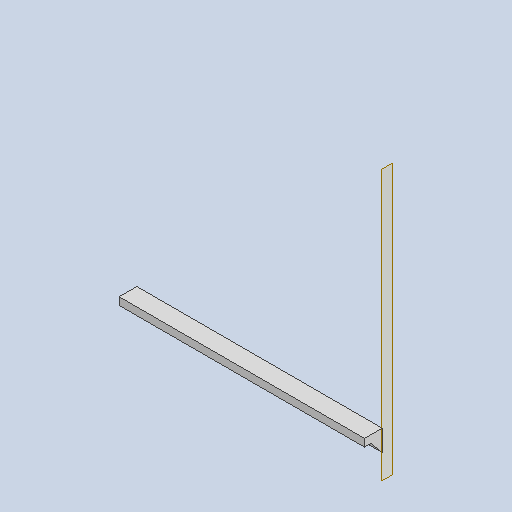
# Autodesk Inventor part: PlasticBody
Saved by Autodesk Inventor 2023 (Build 270158000, 158)
## iProperties
Created: 2024-03-04
Part Number: PlasticBody
Material: Generic
Document SubType Name: Modeling
Designer: pavel
Density: 1 g/cm^3
Appearance: Default
Author: pavel
Autodesk Inventor part; units mm, degrees
ref_plane "YZ Plane" through (0, 0, 0) normal (1, 0, 0) x (0, 1, 0)
ref_plane "XZ Plane" through (0, 0, 0) normal (0, 1, 0) x (-1, 0, 0)
ref_plane "Work Plane1" through (40.8257, 10.5425, -12.0056) normal (1, 0, 0) x (0, 1, 0)
sketch "Sketch1" plane through (40.8257, 10.5425, -12.0056) normal (1, 0, 0) x (0, 1, 0)
  line L0 (4.767, 4) -> (97, 4) projected
  line L1 (0, 0) -> (97, 0) projected
  line L2 (97, 0) -> (97, 4) projected
  line L3 (4.767, 4) -> (97, 4) projected
  line L4 (0, 0) -> (13.1093, 11)
  line L5 (10.1299, 11) -> (13.1093, 11)
  line L6 (10.1299, 11) -> (10.1299, 8.5)
  line L7 (13.1093, 11) -> (13.1093, 4)
  line L8 (4.767, 4) -> (13.1093, 4)
  line L9 (4.767, 4) -> (0, 0) projected
  point P0 (-10.5425, 12.0056)
  point P1 (4.767, 4)
  dimension "d2" = 7
  dimension "d3" = 40
  dimension "d4" = 2.5
  constraints: 10 end point, 4 point on line, 1 collinear, 1 horizontal, 1 perpendicular, 1 vertical
  measures "d2" distance from line of L4.end L0
  measures "d3" angle of L1 L4
  measures "d4" distance of L5.start L6.end
ref_plane "Work Plane2" through (-56.1743, 10.5425, -12.0056) normal (-1, 0, 0) x (0, 0, 1)
extrude "Extrusion1" add sketch "Sketch1" against normal up to surface (97 mm away) contours L4 L7 L0 | L6 L5 L4
body "Solid1"
